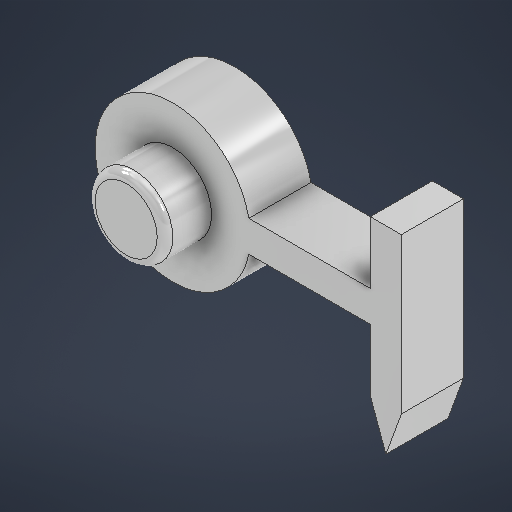
# Autodesk Inventor part: solda
Saved by Autodesk Inventor 2026.4 (Build 304435000, 435)
## iProperties
Created: 2026-08-27
Part Number: solda
Material: Genérico
Document SubType Name: Modeling
Designer: Matheus
Density: 1 g/cm^3
Appearance: Alumínio - Escuro
Author: Matheus
Autodesk Inventor part; units mm, degrees
ref_plane "YZ Plane" through (0, 0, 0) normal (1, 0, 0) x (0, 1, 0)
ref_plane "XZ Plane" through (0, 0, 0) normal (0, 1, 0) x (-1, 0, 0)
ref_plane "XY Plane" through (0, 0, 0) normal (0, 0, 1) x (1, 0, 0)
sketch "Esboço1" plane through (0, 0, 0) normal (0, 0, 1) x (1, 0, 0)
  arc A0 (4.899, 1) -> (4.899, -1) centre (0, 0) ccw
  line L0 (14.72, 0) -> (14.72, 1)
  line L1 (12.72, 1) -> (4.899, 1)
  line L2 (0, 0) -> (14.72, 0) construction
  line L3 (14.72, 0) -> (14.72, -1)
  line L4 (12.7254, -1) -> (4.899, -1)
  line L5 (12.72, 5) -> (14.72, 5)
  line L6 (14.72, 5) -> (14.72, -5)
  line L7 (14.72, -5) -> (12.7254, -5) construction
  line L8 (12.7254, -5) -> (12.7254, -1)
  line L9 (12.72, 1) -> (12.72, 5)
  line L10 (12.7254, -5) -> (13.7254, -7.74)
  line L11 (14.72, -5) -> (13.7254, -7.74)
  dimension "d9" = 10
  dimension "d10" = 1
  dimension "d11" = 1
  dimension "d13" = 2
  dimension "d14" = 10
  dimension "d15" = 4
  dimension "d16" = 4
  dimension "d18" = 40
  dimension "d19" = 2.74
  constraints: 24 end point, 4 parallel, 2 horizontal, 2 perpendicular, 2 point on circle, 2 point on line, 1 centre point, 1 coincident
  measures "d9" diameter of A0
  measures "d10" distance of L0.start L0.end
  measures "d11" distance of L2.end L3.end
  measures "d13" distance of L5.start L5.end
  measures "d14" distance of L5.end L6.end
  measures "d15" distance of L4.start L7.end
  measures "d16" distance of L1.start L5.start
  measures "d18" angle of L11 L10
  measures "d19" vertical distance of L7.end L10.end
extrude "Extrusão1" add sketch "Esboço1" along normal mid plane 4
sketch "Esboço2" plane through (0, 0, 2) normal (0, 0, 1) x (1, 0, 0)
  circle A0 centre (0, 0) radius 2.5
  dimension "d22" = 5
  constraints: 1 centre point, 1 coincident
  measures "d22" diameter of A0
extrude "Extrusão2" add sketch "Esboço2" along normal blind 3
fillet "Arredondamento1" radius 0.5 1 edges at (-2.5, 0, 5)
